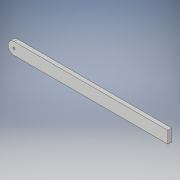
# Autodesk Inventor part: Wheel Arms
Saved by Autodesk Inventor 2019 (Build 230136000, 136)
## iProperties
Created: 2019-10-05
Part Number: Wheel Arms
Material: Generic
Document SubType Name: Modeling
Designer: Delta
Density: 1 g/cm^3
Appearance: Default
Author: Delta
Autodesk Inventor part; units mm, degrees
ref_plane "YZ Plane" through (0, 0, 0) normal (1, 0, 0) x (0, 1, 0)
ref_plane "XZ Plane" through (0, 0, 0) normal (0, 1, 0) x (-1, 0, 0)
ref_plane "XY Plane" through (0, 0, 0) normal (0, 0, 1) x (1, 0, 0)
sketch "Sketch1" plane through (0, 0, 0) normal (0, 0, 1) x (1, 0, 0)
  line L0 (0, 0) -> (254, 0)
  line L1 (254, 0) -> (254, -19.05)
  line L2 (254, -19.05) -> (0, -19.05)
  line L3 (0, -19.05) -> (0, 0)
  dimension "d0" = 254
  dimension "d1" = 19.05
  constraints: 8 end point, 2 parallel, 1 horizontal, 1 perpendicular
  measures "d0" distance of L1.end L2.end
  measures "d1" distance of L0.end L1.end
extrude "Extrusion1" add sketch "Sketch1" along normal blind 6.35
fillet "Fillet1" radius 9.525 2 edges at (0, -19.05, 3.175) (0, 0, 3.175)
sketch "Sketch4" plane through (0, 0, 6.35) normal (0, 0, 1) x (1, 0, 0)
  arc A0 (9.525, 0) -> (9.525, -19.05) centre (9.525, -9.525) ccw projected
  circle A1 centre (9.525, -9.525) radius 1.778
  point P0 (0, 0)
  point P1 (254, 0)
  point P2 (254, -19.05)
  dimension "d14" = 3.556
  constraints: 1 centre point, 1 coincident, 1 other
  measures "d14" diameter of A1
extrude "Extrusion4" cut sketch "Sketch4" against normal blind 12.7
body "Solid1"
